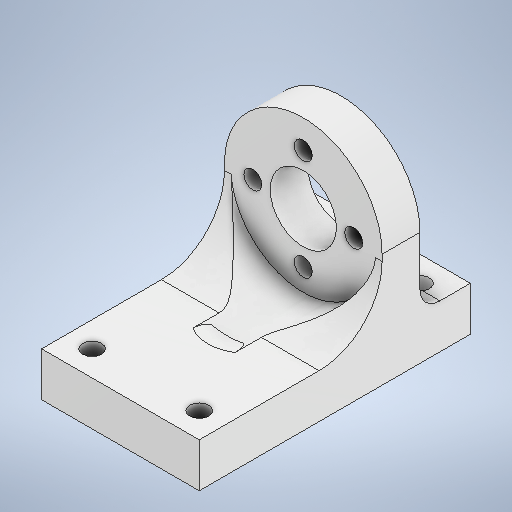
# Autodesk Inventor part: NutMount
Saved by Autodesk Inventor 2026.2 (Build 302298000, 298)
## iProperties
Created: 2026-03-16
Part Number: NutMount
Material: ABS Plastic
Document SubType Name: Modeling
Designer: gaoet
Density: 1.06 g/cm^3
Appearance: Smooth - White
Author: gaoet
Autodesk Inventor part; units mm, degrees
ref_plane "YZ Plane" through (0, 0, 0) normal (1, 0, 0) x (0, 1, 0)
ref_plane "XZ Plane" through (0, 0, 0) normal (0, 1, 0) x (-1, 0, 0)
ref_plane "XY Plane" through (0, 0, 0) normal (0, 0, 1) x (1, 0, 0)
sketch "Sketch1" plane through (0, 0, 0) normal (0, 0, 1) x (1, 0, 0)
  circle A0 centre (0, 0) radius 12.5
  circle A1 centre (0, 0) radius 5.25
  line L0 (12.5, 0) -> (12.5, -18)
  line L1 (12.5, -18) -> (-12.5, -18)
  line L2 (-12.5, -18) -> (-12.5, 0)
  point P0 (-8, 0)
  point P1 (8, 0)
  point P2 (0, 8)
  point P3 (0, -8)
  dimension "d0" = 25
  dimension "d3" = 10.5
  dimension "d4" = 8
  dimension "d5" = 8
  dimension "d13" = 18
  dimension "d73" = 8
  dimension "d74" = 8
  constraints: 6 end point, 2 centre point, 2 coincident, 2 horizontal alignment, 2 point on circle, 2 tangent, 2 vertical, 2 vertical alignment, 1 horizontal
  measures "d0" diameter of A0
  measures "d3" diameter of A1
  measures "d4" distance of point (0, 0) point (8, 0)
  measures "d5" distance of point (0, 0) point (-8, 0)
  measures "d13" distance from line of L1 point (0, 0)
  measures "d73" distance of point (0, 8) point (0, 0)
  measures "d74" distance of point (0, -8) point (0, 0)
extrude "Extrusion1" add sketch "Sketch1" along normal blind 6
hole "Hole1" at (-8, 0, 0) at (8, 0, 0) at (0, 8, 0) at (0, -8, 0) direction (0, 0, 1) diameter 2.85 end through all
sketch "Sketch2" plane through (-12.5, -18, 0) normal (-1, 0, 0) x (0, 0, 1)
  line L0 (0, 18) -> (0, 0) projected
  line L1 (0, 0) -> (6, 0) projected
  line L2 (6, 18) -> (6, 0) projected
  line L3 (0, 18) -> (6, 18) projected
  line L4 (6, 0) -> (35, 0)
  line L5 (35, 0) -> (35, 7)
  line L6 (35, 7) -> (6, 7)
  line L7 (0, 7) -> (-8, 7)
  line L8 (-8, 7) -> (-8, 0)
  line L9 (-8, 0) -> (0, 0)
  point P0 (0, 18)
  dimension "d14" = 7
  dimension "d15" = 35
  dimension "d18" = 8
  constraints: 12 end point, 3 horizontal, 3 perpendicular, 2 point on line, 1 horizontal alignment
  measures "d14" distance of L4.end L5.end
  measures "d15" distance between parallel lines of L0 L5
  measures "d18" distance from line of L0.end L8
extrude "Extrusion2" add sketch "Sketch2" against normal up to surface (25 mm away) contours L0 L9 L8 L7 | L6 L5 L4 L2
sketch "Sketch11" plane through (0, 0, 0) normal (1, 0, 0) x (0, 1, 0)
  line L0 (-11, 0) -> (-11, -8) projected
  line L1 (12.5, 0) -> (0, 0) projected
  line L2 (-11, -8) -> (12.5, 0)
  line L3 (0, 0) -> (0, 0) projected
  line L4 (0, 0) -> (0, 6) projected
  line L5 (0, 6) -> (0, 6) projected
  line L6 (0, 0) -> (0, 6) projected
  line L7 (-11, 35) -> (-11, 6) projected
  line L8 (0, 6) -> (-11, 6) projected
  line L9 (0, 0) -> (0, 6) projected
  line L10 (0, 0) -> (-11, 0) projected
  line L11 (-11, 0) -> (-11, -8) projected
  line L12 (-18, -8) -> (-18, 35) projected
  line L13 (0, -4.2553) -> (0, 0)
  line L14 (-11, -8) -> (-18, -8) projected
  line L15 (-18, 35) -> (-11, 35) projected
  constraints: 4 end point, 1 point on line, 1 vertical
extrude "Extrusion10" [suppressed]
sketch "Sketch13" plane through (-12.5, -18, -8) normal (0, 0, -1) x (-1, 0, 0)
  line L0 (-25, 7) -> (-25, 0) projected
  line L1 (0, 0) -> (-25, 0) projected
  line L2 (0, 7) -> (0, 0) projected
  line L3 (0, 7) -> (-25, 7) projected
  line L4 (0, 18) -> (0, 7) projected
  arc A0 (0, 18) -> (-25, 18) centre (-12.5, 18) ccw projected
  line L5 (-25, 7) -> (-25, 18) projected
  circle A1 centre (-12.5, 18) radius 5.25 projected
  circle A2 centre (-4.5, 18) radius 1.425 projected
  circle A3 centre (-20.5, 18) radius 1.425 projected
  circle A4 centre (-12.5, 18) radius 11.5
  line L6 (-25, 7) -> (0, 7) projected
  point P0 (-15.8541, 7)
  point P1 (-9.1459, 7)
  dimension "d64" = 23
  constraints: 1 centre point, 1 coincident
  measures "d64" diameter of A4
extrude "Extrusion12" cut sketch "Sketch13" against normal up to surface (8 mm away) contours L3 A4 picked at (-12.8776, 6.852)
fillet "Fillet3" radius 3.175 5 edges at (-7.9271, -11, 0) (7.9271, -11, 0) (0, -11.5, 0) (-3.3541, -11, -4) (3.3541, -11, -4)
sketch "Sketch14" plane through (0, 0, 6) normal (0, 0, 1) x (1, 0, 0)
  line L0 (-12.5, -11) -> (12.5, -11) projected
  line L1 (12.5, -11) -> (12.5, 0) projected
  arc A0 (12.5, 0) -> (-12.5, 0) centre (0, 0) ccw projected
  line L2 (-12.5, 0) -> (-12.5, -11) projected
  circle A1 centre (8, 0) radius 1.425 projected
  circle A2 centre (-8, 0) radius 1.425 projected
  circle A3 centre (0, 0) radius 5.25 projected
  circle A4 centre (0, 0) radius 11.5
  point P0 (-11.5, 0)
  point P1 (11.5, 0)
  point P2 (3.3541, -11)
  point P3 (-3.3541, -11)
  dimension "d68" = 23
  constraints: 1 centre point, 1 coincident
  measures "d68" diameter of A4
extrude "Extrusion13" cut sketch "Sketch14" along normal blind 12 contours A4 L0 | L0 A4
fillet "Fillet4" radius 10 2 edges at (7.9271, -11, 6) (-7.9271, -11, 6)
fillet "Fillet5" radius 10 1 edges at (0, -11, 18)
sketch "Sketch15" plane through (-12.5, -18, 35) normal (0, -1, 0) x (1, 0, 0)
  line L0 (21, -4) -> (4, -4)
  line L1 (4, -4) -> (4, -39)
  line L2 (4, -39) -> (21, -39)
  line L3 (21, -39) -> (21, -4)
  line L4 (0, -43) -> (25, -43) projected
  line L5 (0, 0) -> (25, 0) projected
  line L6 (25, -43) -> (25, 0) projected
  line L7 (0, -43) -> (0, 0) projected
  point P0 (12.5, -35)
  point P1 (12.5, -43)
  dimension "d75" = 4
  dimension "d76" = 4
  dimension "d77" = 4
  dimension "d78" = 4
  constraints: 8 end point, 2 parallel, 1 horizontal, 1 midpoint, 1 perpendicular
  measures "d75" distance from line of point (12.5, -43) L2
  measures "d76" distance between parallel lines of L5 L0
  measures "d77" distance between parallel lines of L6 L3
  measures "d78" distance between parallel lines of L7 L1
hole "Hole3" at (-8.5, -18, -4) at (8.5, -18, -4) at (8.5, -18, 31) at (-8.5, -18, 31) direction (0, 1, 0) diameter 3 end through all
equation "\"d4\" = d5"
equation "\"d73\" = d5"
equation "\"d74\" = d73"
body "Solid1"
